DHEC proto sensor v1 (Autodesk Fusion 360 design; units mm, degrees)
Autodesk Fusion 360 part; units mm, degrees
sketch "Sketch1" plane through (0, 0, 0) normal (0, 0, 1) x (1, 0, 0)
  circle A0 centre (0, 0) radius 38.1
  circle A1 centre (0, 0) radius 37.1
  line L0 (24.903, -27.5) -> (24.903, 27.5)
  line L1 (26.903, -25.5468) -> (26.903, 25.5468)
  line L2 (26.903, 12.5) -> (28.903, 12.5)
  line L3 (28.903, 12.5) -> (28.903, -12.5)
  line L4 (28.903, -12.5) -> (26.903, -12.5)
  line L5 (26.903, -12.5) -> (26.903, 12.5)
  line L6 (26.903, 14.5) -> (30.903, 14.5)
  line L7 (30.903, 14.5) -> (30.903, 9.5)
  line L8 (30.903, 9.5) -> (28.903, 9.5)
  line L9 (26.903, -14.5) -> (30.903, -14.5)
  line L10 (30.903, -14.5) -> (30.903, -9.5)
  line L11 (30.903, -9.5) -> (28.903, -9.5)
  line L12 (1.75, 0) -> (22.5, 0)
  line L13 (24.903, 26.75) -> (22.903, 26.75)
  line L14 (22.903, 26.75) -> (22.903, -26.75)
  line L15 (22.903, -26.75) -> (24.903, -26.75)
  line L16 (24.903, -26.75) -> (24.903, 26.75)
  line L17 (22.903, 18.08) -> (11.903, 18.08)
  line L18 (11.903, 18.08) -> (11.903, 5.58)
  line L19 (11.903, 5.58) -> (22.903, 5.58)
  line L20 (22.903, 5.58) -> (22.903, 18.08)
  line L21 (22.903, -13.25) -> (11.903, -13.25)
  line L22 (11.903, -13.25) -> (11.903, -22.5)
  line L23 (11.903, -22.5) -> (22.903, -22.5)
  line L24 (22.903, -22.5) -> (22.903, -13.25)
  line L25 (30.903, -9.5) -> (30.903, 9.5)
  line L26 (0, -38.1) -> (0, 38.1) construction
  line L27 (-38.1, 0) -> (38.1, 0) construction
  line L28 (26.9408, -26.9408) -> (-26.9408, 26.9408) construction
  line L29 (26.9408, 26.9408) -> (-26.9408, -26.9408) construction
  line L30 (0, 37.1) -> (0, 38.1)
  line L31 (-26.2337, 26.2337) -> (-26.9408, 26.9408)
  line L32 (-37.1, 0) -> (-38.1, 0)
  line L33 (-26.9408, -26.9408) -> (-26.2337, -26.2337)
  line L34 (0, -38.1) -> (0, -37.1)
  line L35 (26.9408, -26.9408) -> (26.2337, -26.2337)
  line L36 (38.1, 0) -> (37.1, 0)
  line L37 (26.9408, 26.9408) -> (26.2337, 26.2337)
  line L38 (20.903, 30.6508) -> (20.903, 20.08)
  line L39 (20.903, 20.08) -> (9.903, 20.08)
  line L40 (9.903, 20.08) -> (9.903, 3.58)
  line L41 (9.903, 3.58) -> (22.903, 3.58)
  point P0 (28.903, 0)
  point P1 (22.903, 0)
  dimension "d1" = 76.2
  dimension "d2" = 1
  dimension "d3" = 55
  dimension "d4" = 2
  dimension "d5" = 2
  dimension "d6" = 2
  dimension "d7" = 2
  dimension "d8" = 3
  dimension "d9" = 25
  dimension "d10" = 2
  dimension "d11" = 2
  dimension "d12" = 53.5
  dimension "d13" = 12.5
  dimension "d14" = 11
  dimension "d15" = 8.67
  dimension "d16" = 9.25
  dimension "d17" = 11
  dimension "d18" = 4.25
  dimension "d23" = 45
  dimension "d27" = 2
  dimension "d28" = 2
  dimension "d29" = 2
  dimension "d30" = 2
  constraint coincident A0.centre A1.centre
  constraint coincident A1 L0.start
  constraint coincident A1 L0.end
  constraint vertical L0
  constraint coincident A1 L1.start
  constraint coincident A1 L1.end
  constraint parallel L0 L1
  constraint horizontal L2
  constraint vertical L3
  constraint horizontal L4
  constraint vertical L5
  constraint coincident L1 L2.start
  constraint coincident L1 L6.start
  constraint perpendicular L1 L6
  constraint perpendicular L6 L7
  constraint coincident L3 L8.end
  constraint perpendicular L3 L8
  constraint coincident L1 L9.start
  constraint perpendicular L1 L9
  constraint perpendicular L9 L10
  constraint coincident L3 L11.end
  constraint perpendicular L3 L11
  constraint equal L6 L9
  constraint equal L7 L10
  constraint midpoint L3 P0
  constraint coincident P0 L12
  constraint horizontal L13
  constraint vertical L14
  constraint horizontal L15
  constraint vertical L16
  constraint coincident L0 L13.start
  constraint midpoint L14 P1
  constraint coincident L12 P1
  constraint horizontal L17
  constraint vertical L18
  constraint horizontal L19
  constraint vertical L20
  constraint coincident L14 L17.start
  constraint horizontal L21
  constraint vertical L22
  constraint horizontal L23
  constraint vertical L24
  constraint coincident L14 L21.start
  constraint coincident A0 L26.start
  constraint coincident A0 L26.end
  constraint vertical L26
  constraint coincident A0 L27.start
  constraint coincident A0 L27.end
  constraint perpendicular L3 L27
  constraint coincident A0 L28.start
  constraint coincident A0 L28.end
  constraint coincident A0 L29.start
  constraint coincident A0 L29.end
  constraint coincident A0.centre L29
  constraint coincident A0.centre L28
  constraint coincident A0.centre L26
  constraint coincident A0.centre L27
  constraint perpendicular L28 L29
  constraint coincident L26 L30.start
  constraint coincident A1 L30.start
  constraint coincident A1 L31.start
  constraint coincident L28 L31.start
  constraint coincident A1 L32.start
  constraint coincident L27 L32.start
  constraint coincident L29 L33.end
  constraint coincident A1 L33.end
  constraint coincident A1 L34.end
  constraint coincident L26 L34.end
  constraint coincident L28 L35.end
  constraint coincident A1 L35.end
  constraint coincident A1 L36.end
  constraint coincident L27 L36.end
  constraint coincident A1 L37.end
  constraint coincident L29 L37.end
  constraint perpendicular L38 L39
  constraint coincident L14 L41.end
  constraint perpendicular L14 L41
  constraint coincident A1 L38.start
  measures "d1" diameter of A0
  measures "d2" distance of A0 A1
  measures "d3" distance of L0.start L0.end
  measures "d4" distance of L0 L1
  measures "d5" distance of L3 L5
  measures "d6" distance of L4 L9
  measures "d7" distance of L3 L10
  measures "d8" distance of L4 L11
  measures "d9" distance of L2 L4
  measures "d10" distance of L2 L6
  measures "d11" distance of L0 L14
  measures "d12" distance of L13.end L14.end
  measures "d13" distance of L17 L19
  measures "d14" distance of L18 L20
  measures "d15" distance of L13.end L17
  measures "d16" distance of L21 L23
  measures "d17" distance of L14 L22
  measures "d18" distance of L15 L23
  measures "d23" angle of L27 L28
  measures "d27" distance of L18 L40
  measures "d28" distance of L17 L39
  measures "d29" distance of L19 L41
  measures "d30" distance of L14 L38
extrude "Extrude1" add sketch "Sketch1" along normal blind 2 contours A1 L1 L6 L7 L9 L10 L25 | A1 L0 L14 L15 L21 L22 L23 L38 L39 L40 L41 | A1 L0 L13 L14 L17 L18 L19 L38 L39 L40 L41 | L0 L13 L14 L15 L16 L20 L24 makes body 1 at (-3.5853, -7.0522, 0) makes body 2 at (32.7043, -2.5435, 0)
extrude "Extrude2" add sketch "Sketch1" along normal blind 15 contours L1 L2 L3 L6 L7 L8 | L1 L3 L4 L9 L10 L11 bodies 2
extrude "Extrude3" add sketch "Sketch1" along normal blind 120 contours A0 A1 L35 L36 | A0 A1 L30 L37 | A1 L0 L1 L5 L16 | A0 A1 L33 L34 | A0 A1 L31 L32 bodies 2 1
extrude "Extrude4" add sketch "Sketch1" along normal blind 10 contours A1 L0 L13 L14 L17 L18 L19 L38 L39 L40 L41 bodies 2
